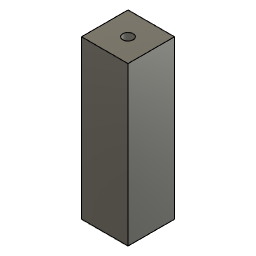
Assembly (Autodesk Fusion 360 archive; units mm, degrees)
design "15*15"
Autodesk Fusion 360 part; units mm, degrees
sketch "Sketch1" plane through (0, 0, 0) normal (0, 1, 0) x (1, 0, 0)
  line L0 (-7.5, 7.5) -> (7.5, 7.5)
  line L1 (-7.5, -7.5) -> (7.5, 7.5) construction
  line L2 (7.5, 7.5) -> (7.5, -7.5)
  circle A0 centre (0, 0) radius 1.7
  line L3 (7.5, -7.5) -> (-7.5, -7.5)
  line L4 (7.5, -7.5) -> (-7.5, 7.5) construction
  line L5 (-7.5, -7.5) -> (-7.5, 7.5)
  dimension "d1" = 15
  dimension "d2" = 15
  dimension "d3" = 3.4
  constraint horizontal L3
  constraint perpendicular L3 L5
  constraint parallel L0 L3
  constraint parallel L2 L5
  constraint coincident A0.centre L4
  constraint coincident A0.centre L1
  constraint coincident A0.centre origin
  measures "d1" distance of L0.start L0.end
  measures "d2" distance of L1.start L0.start
  measures "d3" diameter of A0
extrude "Extrude1" add sketch "Sketch1" along normal blind 5
sketch "Sketch2" plane through (0, 5, 0) normal (0, 1, 0) x (-1, 0, 0)
  circle A0 centre (0, 0) radius 1.7
  line L0 (7.5, 7.5) -> (-7.5, 7.5)
  line L1 (-7.5, 7.5) -> (-7.5, -7.5)
  line L2 (-7.5, -7.5) -> (7.5, -7.5)
  line L3 (7.5, -7.5) -> (7.5, 7.5)
  line L4 (-3.3486, -3.4) -> (-3.3486, 0)
  line L5 (-1.6743, 2.9) -> (-3.3486, 0)
  line L6 (1.6743, 2.9) -> (-1.6743, 2.9)
  circle A1 centre (0, 0) radius 1.7
  line L7 (3.3486, 0) -> (3.3486, -3.1)
  line L8 (3.3486, 0) -> (1.6743, 2.9)
  line L9 (3.3486, -3.1) -> (3.3486, -3.4)
  line L10 (3.3486, -3.4) -> (3.3486, -7.5)
  line L11 (-3.3486, -3.4) -> (-3.3486, -7.5)
  line L12 (3.3486, -7.5) -> (-3.3486, -7.5)
  point P0 (0, 0.15)
  point P1 (0, 0.15)
  dimension "d6" = 2.75
  dimension "d16" = 0.3
  constraint coincident P1 P0
  constraint coincident L2 L10.end
  constraint perpendicular L2 L10
  constraint coincident L2 L11.end
  constraint perpendicular L2 L11
  measures "d6" distance of P1 L6
  measures "d16" distance of L9.end L7.end
extrude "Extrude2" add sketch "Sketch2" along normal blind 4.5 contours L0 L1 L2 L3 L4 L5 L6 L7 L8 L9 L10 L11
sketch "Sketch3" plane through (0, 9.5, 0) normal (0, 1, 0) x (-1, 0, 0)
  line L0 (1.6743, 2.9) -> (3.3486, 0)
  line L1 (3.3486, 0) -> (3.3486, -7.5)
  line L2 (-3.3486, -7.5) -> (-3.3486, 0)
  line L3 (-3.3486, 0) -> (-1.6743, 2.9)
  line L4 (-1.6743, 2.9) -> (1.6743, 2.9)
  line L5 (7.5, -7.5) -> (7.5, 7.5)
  line L6 (7.5, 7.5) -> (-7.5, 7.5)
  line L7 (-7.5, 7.5) -> (-7.5, -7.5)
  line L8 (3.3486, -7.5) -> (7.5, -7.5)
  line L9 (7.5, -7.5) -> (-7.5, -7.5)
  line L10 (-7.5, -7.5) -> (-7.5, 7.5)
  line L11 (-7.5, 7.5) -> (7.5, 7.5)
  line L12 (7.5, 7.5) -> (7.5, -7.5)
  circle A0 centre (0, 0) radius 1.65
  line L13 (-7.5, -7.5) -> (-3.3486, -7.5)
  dimension "d12" = 3.3
  constraint horizontal L9
  constraint vertical L10
  constraint horizontal L11
  constraint vertical L12
  constraint coincident L6.end L7.start
  constraint coincident L5.start L8.end
  constraint coincident A0.centre origin
  measures "d12" diameter of A0
extrude "Extrude3" add sketch "Sketch3" along normal blind 5
sketch "Sketch4" plane through (0, 14.5, 0) normal (0, 1, 0) x (-1, 0, 0)
  circle A0 centre (0, 0) radius 1.65
  line L0 (7.5, 7.5) -> (-7.5, 7.5)
  line L1 (-7.5, 7.5) -> (-7.5, -7.5)
  line L2 (-7.5, -7.5) -> (7.5, -7.5)
  line L3 (7.5, -7.5) -> (7.5, 7.5)
  line L4 (7.5, -7.5) -> (-7.5, -7.5)
  line L5 (-7.5, -7.5) -> (-7.5, 7.5)
  line L6 (-7.5, 7.5) -> (7.5, 7.5)
  line L7 (7.5, 7.5) -> (7.5, -7.5)
  constraint horizontal L4
  constraint vertical L5
  constraint horizontal L6
  constraint vertical L7
  constraint coincident L0.end L1.start
  constraint coincident L2.end L3.start
extrude "Extrude4" add sketch "Sketch4" along normal blind 11 contours A0 | L0 L1 L2 L3 L4 L5 L6 L7
mirror "Mirror1" about plane through (0, 25.5, 0) normal (0, 1, 0) of bodies 1 merged
equation "d6 = ( 5.5 / 2 ) * 1 mm"
equation "d13 = 2.5 mm + 8.5 mm"

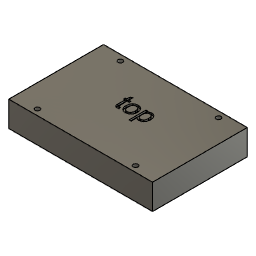
design "RPI"
Autodesk Fusion 360 part; units mm, degrees
sketch "Sketch1" plane through (0, 0, 0) normal (0, 1, 0) x (1, 0, 0)
  line L0 (42.5, -28) -> (-42.5, -28)
  line L1 (-42.5, -28) -> (-42.5, 28)
  line L2 (-42.5, 28) -> (42.5, 28)
  line L3 (42.5, 28) -> (42.5, -28)
  line L4 (42.5, -28) -> (-42.5, 28) construction
  line L5 (-42.5, -28) -> (42.5, 28) construction
  line L6 (0, 28) -> (29, 28)
  line L7 (29, 28) -> (29, -28)
  line L8 (29, 0) -> (29, 24.5)
  line L9 (29, 0) -> (29, -24.5)
  line L10 (29, 24.5) -> (-29, 24.5)
  line L11 (29, -24.5) -> (-29, -24.5)
  circle A0 centre (-29, 24.5) radius 1.4
  circle A1 centre (-29, -24.5) radius 1.4
  circle A2 centre (29, -24.5) radius 1.4
  circle A3 centre (29, 24.5) radius 1.4
  dimension "d1" = 85
  dimension "d2" = 56
  dimension "d3" = 29
  dimension "d4" = 24.5
  dimension "d5" = 24.5
  dimension "d6" = 58
  dimension "d7" = 58
  dimension "d8" = 2.8
  dimension "d9" = 2.8
  dimension "d10" = 2.8
  dimension "d11" = 2.8
  constraint horizontal L0
  constraint perpendicular L0 L1
  constraint parallel L0 L2
  constraint parallel L1 L3
  constraint coincident L4 origin
  constraint coincident L5 origin
  constraint midpoint L2 L6.start
  constraint parallel L2 L6
  constraint coincident L0 L7.end
  constraint perpendicular L0 L7
  constraint midpoint L7 L8.start
  constraint perpendicular L6 L8
  constraint perpendicular L2 L9
  constraint perpendicular L7 L10
  constraint perpendicular L9 L11
  constraint coincident L10.end A0.centre
  constraint coincident L11.end A1.centre
  constraint coincident L9.end L11.start
  constraint coincident L8.end L10.start
  measures "d1" distance of L1.end L2.end
  measures "d2" distance of L0.end L1.end
  measures "d3" distance of L6.start L6.end
  measures "d4" distance of L8.start L8.end
  measures "d5" distance of L8.start L9.end
  measures "d6" distance of L8.end L10.end
  measures "d7" distance of L9.end L11.end
  measures "d8" diameter of A0
  measures "d9" diameter of A1
  measures "d10" diameter of A2
  measures "d11" diameter of A3
extrude "Extrude1" add sketch "Sketch1" along normal blind 15 contours L0 L2 L3 L7 L8 L9 A2 A3 | L0 L1 L2 L6 L7 L8 L9 A2 A3
sketch "Sketch2" plane through (0, 15, 0) normal (0, 1, 0) x (-1, 0, 0)
  circle A0 centre (-29, -24.5) radius 1.4
  circle A1 centre (-29, 24.5) radius 1.4
  circle A2 centre (29, -24.5) radius 1.4
  circle A3 centre (29, 24.5) radius 1.4
  line L0 (-42.5, -28) -> (42.5, -28)
  line L1 (42.5, -28) -> (42.5, 28)
  line L2 (42.5, 28) -> (-42.5, 28)
  line L3 (-42.5, 28) -> (-42.5, -28)
  line L4 (8.6608, -1) -> (-5, -1) construction
  line L5 (-5, -1) -> (-5, -9.5323) construction
  line L6 (-5, -9.5323) -> (8.6608, -9.5323) construction
  line L7 (8.6608, -9.5323) -> (8.6608, -1) construction
  dimension "d14" = 10
  text T0 "top" font "Arial" height 10 align left top in box 13.6608 x 8.5323 at (8.6608, -1) x (-1, 0) y (0, -1) spacing 1 kerned
extrude "Extrude2" cut sketch "Sketch2" against normal blind 1 text T0
equation "d3 = ( 58 / 2 ) * 1 mm"
equation "d4 = ( 49 / 2 ) * 1 mm"
equation "d5 = ( 49 / 2 ) * 1 mm"

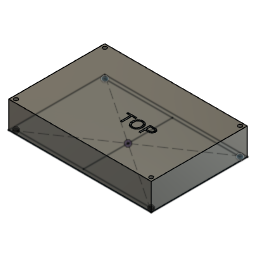
design "AMP"
Autodesk Fusion 360 part; units mm, degrees
sketch "Sketch1" plane through (0, 0, 0) normal (0, 1, 0) x (1, 0, 0)
  line L0 (64.05, -43.15) -> (-64.05, -43.15)
  line L1 (-64.05, -43.15) -> (-64.05, 43.15)
  line L2 (-64.05, 43.15) -> (64.05, 43.15)
  line L3 (64.05, 43.15) -> (64.05, -43.15)
  line L4 (64.05, -43.15) -> (-64.05, 43.15) construction
  line L5 (-64.05, -43.15) -> (64.05, 43.15) construction
  line L6 (-59.3743, 40) -> (-60.75, 40)
  line L7 (59.3743, 40) -> (60.75, 40)
  line L8 (0, 0) -> (0, 39.9)
  line L9 (0, 39.9) -> (60.75, 39.9)
  line L10 (0, 39.9) -> (-60.75, 39.9)
  line L11 (0, 0) -> (0, -39.9)
  line L12 (0, -39.9) -> (-60.75, -39.9)
  line L13 (0, -39.9) -> (60.75, -39.9)
  circle A0 centre (-60.75, -39.9) radius 1.65
  circle A1 centre (60.75, -39.9) radius 1.65
  circle A2 centre (60.75, 40) radius 1.65
  circle A3 centre (-60.75, 40) radius 1.65
  dimension "d1" = 128.1
  dimension "d2" = 86.3
  dimension "d5" = 39.9
  dimension "d6" = 60.75
  dimension "d7" = 60.75
  dimension "d8" = 39.9
  dimension "d9" = 60.75
  dimension "d10" = 60.75
  dimension "d11" = 3.3
  dimension "d12" = 3.3
  dimension "d13" = 3.3
  dimension "d14" = 3.3
  constraint horizontal L0
  constraint perpendicular L0 L1
  constraint parallel L0 L2
  constraint parallel L1 L3
  constraint coincident L4 L8.start
  constraint coincident L5 L8.start
  constraint coincident L8.start L11.start
  constraint parallel L2 L6
  constraint parallel L6 L7
  constraint vertical L8
  constraint perpendicular L8 L9
  constraint perpendicular L8 L10
  constraint coincident L4 L6.start
  constraint coincident L5 L7.start
  constraint vertical L11
  constraint perpendicular L11 L12
  constraint perpendicular L11 L13
  constraint coincident L12.end A0.centre
  constraint coincident L13.end A1.centre
  constraint coincident L7.end A2.centre
  constraint coincident L6.end A3.centre
  measures "d1" distance of L1.end L2.end
  measures "d2" distance of L0.end L1.end
  measures "d5" distance of L8.start L8.end
  measures "d6" distance of L8.end L9.end
  measures "d7" distance of L8.end L10.end
  measures "d8" distance of L8.start L11.end
  measures "d9" distance of L11.end L12.end
  measures "d10" distance of L11.end L13.end
  measures "d11" diameter of A0
  measures "d12" diameter of A1
  measures "d13" diameter of A2
  measures "d14" diameter of A3
extrude "Extrude1" add sketch "Sketch1" along normal blind 24
sketch "Sketch2" plane through (0, 24, 0) normal (0, 1, 0) x (-1, 0, 0)
  circle A0 centre (60.75, 39.9) radius 1.65
  circle A1 centre (-60.75, -40) radius 1.65
  circle A2 centre (-60.75, 39.9) radius 1.65
  circle A3 centre (60.75, -40) radius 1.65
  line L0 (-64.05, -43.15) -> (64.05, -43.15)
  line L1 (64.05, -43.15) -> (64.05, 43.15)
  line L2 (64.05, 43.15) -> (-64.05, 43.15)
  line L3 (-64.05, 43.15) -> (-64.05, -43.15)
  line L4 (0, 15.5213) -> (-15.9408, 15.5213) construction
  line L5 (-15.9408, 15.5213) -> (-15.9408, 0) construction
  line L6 (-15.9408, 0) -> (0, 0) construction
  line L7 (0, 0) -> (0, 15.5213) construction
  dimension "d17" = 10
  text T0 "TOP" font "Arial" height 10 align left top in box 15.9408 x 15.5213 at (0, 15.5213) x (-1, 0) y (0, -1) spacing 1 kerned
  constraint coincident L6.end
extrude "Extrude2" cut sketch "Sketch2" against normal blind 2 text T0
equation "d5 = ( 79.8 / 2 ) * 1 mm"
equation "d8 = ( 79.8 / 2 ) * 1 mm"

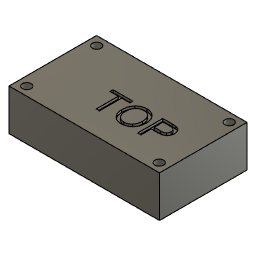
design "Timer relay"
Autodesk Fusion 360 part; units mm, degrees
sketch "Sketch1" plane through (0, 0, 0) normal (0, 1, 0) x (1, 0, 0)
  line L0 (30.1, -17.5) -> (-30.1, -17.5)
  line L1 (-30.1, -17.5) -> (-30.1, 17.5)
  line L2 (-30.1, 17.5) -> (30.1, 17.5)
  line L3 (30.1, 17.5) -> (30.1, -17.5)
  line L4 (30.1, -17.5) -> (-30.1, 17.5) construction
  line L5 (-30.1, -17.5) -> (30.1, 17.5) construction
  line L6 (0, 17.5) -> (-26.5, 17.5)
  line L7 (0, 17.5) -> (26.5, 17.5)
  line L8 (-26.5, 17.5) -> (-26.5, -17.5)
  line L9 (26.5, 17.5) -> (26.5, -17.5)
  line L10 (-26.5, 0) -> (-26.5, 14)
  line L11 (-26.5, 0) -> (-26.5, -14)
  line L12 (26.5, 0) -> (26.5, 14)
  line L13 (26.5, 0) -> (26.5, -14)
  circle A0 centre (-26.5, 14) radius 1.75
  circle A1 centre (26.5, 14) radius 1.75
  circle A2 centre (-26.5, -14) radius 1.75
  circle A3 centre (26.5, -14) radius 1.75
  dimension "d1" = 60.2
  dimension "d2" = 35
  dimension "d3" = 26.5
  dimension "d4" = 26.5
  dimension "d5" = 14
  dimension "d6" = 14
  dimension "d7" = 14
  dimension "d8" = 14
  dimension "d9" = 3.5
  dimension "d10" = 3.5
  dimension "d11" = 3.5
  dimension "d12" = 3.5
  constraint horizontal L0
  constraint perpendicular L0 L1
  constraint parallel L0 L2
  constraint parallel L1 L3
  constraint coincident L4 origin
  constraint coincident L5 origin
  constraint midpoint L2 L6.start
  constraint parallel L2 L6
  constraint parallel L2 L7
  constraint coincident L0 L8.end
  constraint perpendicular L0 L8
  constraint coincident L0 L9.end
  constraint perpendicular L0 L9
  constraint midpoint L8 L10.start
  constraint perpendicular L0 L10
  constraint parallel L8 L11
  constraint midpoint L9 L12.start
  constraint parallel L9 L12
  constraint parallel L9 L13
  constraint coincident L10.end A0.centre
  constraint coincident L12.end A1.centre
  constraint coincident L11.end A2.centre
  constraint coincident L13.end A3.centre
  measures "d1" distance of L1.end L2.end
  measures "d2" distance of L0.end L1.end
  measures "d3" distance of L6.start L6.end
  measures "d4" distance of L6.start L7.end
  measures "d5" distance of L10.start L10.end
  measures "d6" distance of L10.start L11.end
  measures "d7" distance of L12.start L12.end
  measures "d8" distance of L12.start L13.end
  measures "d9" diameter of A0
  measures "d10" diameter of A1
  measures "d11" diameter of A2
  measures "d12" diameter of A3
extrude "Extrude1" add sketch "Sketch1" along normal blind 16.5 contours L0 L2 L3 L9 L12 L13 A1 A3 | L0 L2 L6 L7 L8 L9 L10 L11 L12 L13 A0 A1 A2 A3 | L0 L1 L2 L8 L10 L11 A0 A2
sketch "Sketch2" plane through (0, 16.5, 0) normal (0, 1, 0) x (-1, 0, 0)
  circle A0 centre (26.5, 14) radius 1.75
  circle A1 centre (26.5, -14) radius 1.75
  circle A2 centre (-26.5, 14) radius 1.75
  circle A3 centre (-26.5, -14) radius 1.75
  line L0 (-30.1, -17.5) -> (30.1, -17.5)
  line L1 (30.1, -17.5) -> (30.1, 17.5)
  line L2 (30.1, 17.5) -> (-30.1, 17.5)
  line L3 (-30.1, 17.5) -> (-30.1, -17.5)
  line L4 (8, 8) -> (-13, 8) construction
  line L5 (-13, 8) -> (-13, -2) construction
  line L6 (-13, -2) -> (8, -2) construction
  line L7 (8, -2) -> (8, 8) construction
  dimension "d15" = 10
  text T0 "TOP" font "Arial" height 10 align left top in box 21 x 10 at (8, 8) x (-1, 0) y (0, -1) spacing 1 kerned
extrude "Extrude2" cut sketch "Sketch2" against normal blind 1 text T0
equation "d3 = ( 53 / 2 ) * 1 mm"
equation "d4 = ( 53 / 2 ) * 1 mm"
equation "d5 = ( 28 / 2 ) * 1 mm"
equation "d6 = ( 28 / 2 ) * 1 mm"
equation "d7 = ( 28 / 2 ) * 1 mm"
equation "d8 = ( 28 / 2 ) * 1 mm"

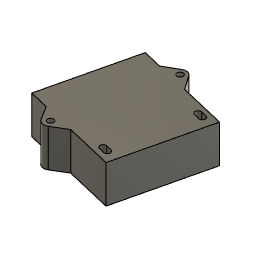
design "buck"
Autodesk Fusion 360 part; units mm, degrees
sketch "Sketch1" plane through (0, 0, 0) normal (0, 1, 0) x (1, 0, 0)
sketch "Sketch2" plane through (0, 0, 0) normal (0, 1, 0) x (1, 0, 0)
  line L0 (-20.092, 27.8314) -> (-31.6, -20.8)
  line L1 (-31.6, -20.8) -> (19.9756, -33.0048)
  line L2 (19.9756, -33.0048) -> (31.4837, 15.6266)
  line L3 (31.4837, 15.6266) -> (-20.092, 27.8314)
  line L4 (24.4539, 11.7249) -> (21.3359, 12.4754)
  line L5 (22.1094, 15.5804) -> (25.144, 14.849)
  arc A0 (22.1094, 15.5804) -> (21.3359, 12.4754) centre (21.7103, 14.031) ccw
  arc A1 (24.3358, 11.7533) -> (25.144, 14.849) centre (24.769, 13.2935) ccw
  arc A2 (14.7267, -28.9815) -> (15.5348, -25.8858) centre (15.1599, -27.4412) ccw
  line L6 (14.8447, -29.0099) -> (11.7267, -28.2593)
  arc A3 (12.5003, -25.1543) -> (11.7267, -28.2593) centre (12.1012, -26.7038) ccw
  line L7 (12.5003, -25.1543) -> (15.5348, -25.8858)
  circle A4 centre (-13.8753, -28.489) radius 1.6
  circle A5 centre (-0.7636, 26.9907) radius 1.6
  line L8 (-10.142, 25.4769) -> (-2.4291, 29.8969)
  line L9 (7.1942, 21.3744) -> (1.9912, 28.8963)
  arc A6 (1.9912, 28.8963) -> (-2.4291, 29.8969) centre (-0.7636, 26.9907) ccw
  line L10 (-21.5261, -23.1839) -> (-17.0355, -30.4438)
  line L11 (-4.4885, -27.2156) -> (-11.9714, -31.6801)
  arc A7 (-17.0355, -30.4438) -> (-11.9714, -31.6801) centre (-13.8753, -28.489) ccw
  dimension "d9" = 53
  dimension "d10" = 3.2
  dimension "d11" = 3.2
  dimension "d12" = 3.2
  dimension "d13" = 3.2
  dimension "d14" = 3.2
  dimension "d15" = 3.2
  constraint perpendicular L0 L1
  constraint parallel L0 L2
  constraint parallel L1 L3
  constraint coincident L4.start A1
  constraint tangent L4 A0
  constraint tangent L5 A1
  constraint coincident L4 A1.start
  constraint coincident L6.start A2
  constraint tangent L6 A3
  constraint tangent A2 L7
  constraint coincident A2.start L6
  constraint coincident L3 L8.start
  constraint coincident L3 L9.start
  constraint concentric A5 A6
  constraint tangent L8 A6
  constraint tangent L9 A6
  constraint coincident L1 L10.start
  constraint coincident L1 L11.start
  constraint concentric A4 A7
  constraint tangent L10 A7
  constraint tangent L11 A7
  measures "d9" distance of L0.start L2.end
  measures "d10" diameter of A0
  measures "d11" diameter of A1
  measures "d12" diameter of A3
  measures "d13" diameter of A2
  measures "d14" diameter of A4
  measures "d15" diameter of A5
extrude "Extrude1" add sketch "Sketch2" along normal blind 20

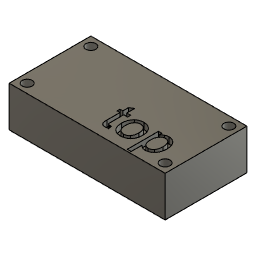
design "Relais"
Autodesk Fusion 360 part; units mm, degrees
sketch "Sketch1" plane through (0, 0, 0) normal (0, 1, 0) x (1, 0, 0)
  line L0 (25.1, -13.15) -> (-25.1, -13.15)
  line L1 (-25.1, -13.15) -> (-25.1, 13.15)
  line L2 (-25.1, 13.15) -> (25.1, 13.15)
  line L3 (25.1, 13.15) -> (25.1, -13.15)
  line L4 (25.1, -13.15) -> (-25.1, 13.15) construction
  line L5 (-25.1, -13.15) -> (25.1, 13.15) construction
  line L6 (0, 0) -> (0, 10.25)
  line L7 (0, 0) -> (0, -10.25)
  line L8 (0, 10.25) -> (-22.2, 10.25)
  line L9 (0, 10.25) -> (22.2, 10.25)
  line L10 (0, -10.25) -> (-22.2, -10.25)
  line L11 (0, -10.25) -> (22.2, -10.25)
  circle A0 centre (-22.2, 10.25) radius 1.6
  circle A1 centre (22.2, 10.25) radius 1.6
  circle A2 centre (-22.2, -10.25) radius 1.6
  circle A3 centre (22.2, -10.25) radius 1.6
  dimension "d1" = 50.2
  dimension "d2" = 26.3
  dimension "d3" = 10.25
  dimension "d4" = 10.25
  dimension "d5" = 22.2
  dimension "d6" = 22.2
  dimension "d7" = 22.2
  dimension "d8" = 22.2
  dimension "d9" = 3.2
  dimension "d10" = 3.2
  dimension "d11" = 3.2
  dimension "d12" = 3.2
  constraint horizontal L0
  constraint perpendicular L0 L1
  constraint parallel L0 L2
  constraint parallel L1 L3
  constraint coincident L4 L6.start
  constraint coincident L5 L6.start
  constraint coincident L6.start L7.start
  constraint perpendicular L2 L6
  constraint parallel L6 L7
  constraint perpendicular L6 L8
  constraint perpendicular L6 L9
  constraint perpendicular L7 L10
  constraint perpendicular L7 L11
  constraint coincident L8.end A0.centre
  constraint coincident L9.end A1.centre
  constraint coincident L10.end A2.centre
  constraint coincident L11.end A3.centre
  measures "d1" distance of L1.end L2.end
  measures "d2" distance of L0.end L1.end
  measures "d3" distance of L6.start L6.end
  measures "d4" distance of L6.start L7.end
  measures "d5" distance of L6.end L8.end
  measures "d6" distance of L6.end L9.end
  measures "d7" distance of L7.end L10.end
  measures "d8" distance of L7.end L11.end
  measures "d9" diameter of A0
  measures "d10" diameter of A1
  measures "d11" diameter of A2
  measures "d12" diameter of A3
extrude "Extrude1" add sketch "Sketch1" along normal blind 13
sketch "Sketch2" plane through (0, 13, 0) normal (0, 1, 0) x (-1, 0, 0)
  circle A0 centre (-22.2, 10.25) radius 1.6
  circle A1 centre (-22.2, -10.25) radius 1.6
  circle A2 centre (22.2, 10.25) radius 1.6
  circle A3 centre (22.2, -10.25) radius 1.6
  line L0 (-25.1, -13.15) -> (25.1, -13.15)
  line L1 (25.1, -13.15) -> (25.1, 13.15)
  line L2 (25.1, 13.15) -> (-25.1, 13.15)
  line L3 (-25.1, 13.15) -> (-25.1, -13.15)
  line L4 (0, 4) -> (-8, 4) construction
  line L5 (-8, 4) -> (-8, 0) construction
  line L6 (-8, 0) -> (0, 0) construction
  line L7 (0, 0) -> (0, 4) construction
  dimension "d15" = 10
  text T0 "top\n" font "Arial" height 10 align left top in box 8 x 4 at (0, 4) x (-1, 0) y (0, -1) spacing 1 kerned
  constraint coincident L6.end
extrude "Extrude2" cut sketch "Sketch2" against normal blind 2 text T0
equation "d3 = ( 20.5 / 2 ) * 1 mm"
equation "d4 = ( 20.5 / 2 ) * 1 mm"
equation "d5 = ( 44.4 / 2 ) * 1 mm"
equation "d6 = ( 44.4 / 2 ) * 1 mm"
equation "d7 = ( 44.4 / 2 ) * 1 mm"
equation "d8 = ( 44.4 / 2 ) * 1 mm"

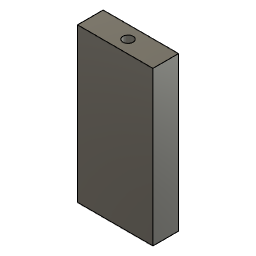
design "20*8.5"
Autodesk Fusion 360 part; units mm, degrees
sketch "Sketch1" plane through (0, 0, 0) normal (0, 1, 0) x (1, 0, 0)
  line L0 (12.5, -4.25) -> (-12.5, -4.25)
  line L1 (-12.5, -4.25) -> (-12.5, 4.25)
  line L2 (-12.5, 4.25) -> (12.5, 4.25)
  line L3 (12.5, 4.25) -> (12.5, -4.25)
  line L4 (12.5, -4.25) -> (-12.5, 4.25) construction
  line L5 (-12.5, -4.25) -> (12.5, 4.25) construction
  circle A0 centre (0, 0) radius 1.7
  dimension "d1" = 25
  dimension "d2" = 8.5
  dimension "d3" = 3.4
  constraint horizontal L0
  constraint perpendicular L0 L1
  constraint parallel L0 L2
  constraint parallel L1 L3
  constraint coincident L4 A0.centre
  constraint coincident L5 A0.centre
  constraint coincident A0.centre origin
  measures "d1" distance of L1.end L2.end
  measures "d2" distance of L0.end L1.end
  measures "d3" diameter of A0
extrude "Extrude1" add sketch "Sketch1" along normal blind 5
sketch "Sketch2" plane through (0, 5, 0) normal (0, 1, 0) x (-1, 0, 0)
  circle A0 centre (0, 0) radius 1.7
  line L0 (-12.5, -4.25) -> (12.5, -4.25)
  line L1 (12.5, -4.25) -> (12.5, 4.25)
  line L2 (12.5, 4.25) -> (-12.5, 4.25)
  line L3 (-12.5, 4.25) -> (-12.5, -4.25)
  line L4 (-1.6743, 2.9) -> (-3.3486, 0)
  line L5 (3.3486, 0) -> (1.6743, 2.9)
  line L6 (1.6743, 2.9) -> (-1.6743, 2.9)
  line L7 (3.3486, 0) -> (3.3486, -2.9)
  line L8 (3.3486, -2.9) -> (3.3486, -3.4)
  line L9 (-3.3486, -3.4) -> (-3.3486, 0)
  line L10 (-3.3486, -3.4) -> (-3.3486, -4.25)
  line L11 (3.3486, -3.4) -> (3.3486, -4.25)
  line L12 (-3.3486, -4.25) -> (3.3486, -4.25)
  dimension "d6" = 2.9
  dimension "d16" = 0.5
  constraint coincident A0.centre origin
  constraint coincident L0 L10.end
  constraint perpendicular L0 L10
  constraint coincident L0 L11.end
  constraint perpendicular L0 L11
  measures "d6" distance of A0.centre L6
  measures "d16" distance of L7.end L8.end
extrude "Extrude2" add sketch "Sketch2" along normal blind 4.5 contours L0 L1 L2 L3 L4 L5 L6 L7 L8 L9 L10 L11
sketch "Sketch3" plane through (0, 9.5, 0) normal (0, 1, 0) x (-1, 0, 0)
  line L0 (-1.6743, 2.9) -> (1.6743, 2.9)
  line L1 (1.6743, 2.9) -> (3.3486, 0)
  line L2 (-3.3486, 0) -> (-1.6743, 2.9)
  line L3 (-12.5, 4.25) -> (-12.5, -4.25)
  line L4 (3.3486, -4.25) -> (12.5, -4.25)
  line L5 (12.5, -4.25) -> (12.5, 4.25)
  line L6 (12.5, 4.25) -> (-12.5, 4.25)
  circle A0 centre (0, 0) radius 1.7
  line L7 (-12.5, 4.25) -> (12.5, 4.25)
  line L8 (12.5, 4.25) -> (12.5, -4.25)
  line L9 (12.5, -4.25) -> (-12.5, -4.25)
  line L10 (-12.5, -4.25) -> (-12.5, 4.25)
  line L11 (-12.5, 4.25) -> (12.5, -4.25) construction
  line L12 (12.5, 4.25) -> (-12.5, -4.25) construction
  line L13 (3.3486, 0) -> (3.3486, -4.25)
  line L14 (-3.3486, -4.25) -> (-3.3486, 0)
  line L15 (-12.5, -4.25) -> (-3.3486, -4.25)
  dimension "d9" = 3.4
  constraint coincident A0.centre origin
  constraint horizontal L7
  constraint perpendicular L7 L8
  constraint parallel L7 L9
  constraint parallel L8 L10
  constraint coincident L11 A0.centre
  constraint coincident L12 A0.centre
  constraint coincident L3.start L6.end
  measures "d9" diameter of A0
extrude "Extrude3" add sketch "Sketch3" along normal blind 5
sketch "Sketch4" plane through (0, 14.5, 0) normal (0, 1, 0) x (-1, 0, 0)
  circle A0 centre (0, 0) radius 1.7
  line L0 (-12.5, -4.25) -> (12.5, -4.25)
  line L1 (12.5, -4.25) -> (12.5, 4.25)
  line L2 (12.5, 4.25) -> (-12.5, 4.25)
  line L3 (-12.5, 4.25) -> (-12.5, -4.25)
  line L4 (-12.5, 4.25) -> (12.5, 4.25)
  line L5 (12.5, 4.25) -> (12.5, -4.25)
  line L6 (12.5, -4.25) -> (-12.5, -4.25)
  line L7 (-12.5, -4.25) -> (-12.5, 4.25)
  line L8 (-12.5, 4.25) -> (12.5, -4.25) construction
  line L9 (12.5, 4.25) -> (-12.5, -4.25) construction
  constraint horizontal L4
  constraint perpendicular L4 L5
  constraint parallel L4 L6
  constraint parallel L5 L7
  constraint coincident L8 A0.centre
  constraint coincident L9 A0.centre
  constraint coincident L2.end L3.start
  constraint coincident A0.centre origin
extrude "Extrude4" add sketch "Sketch4" along normal blind 11 contours A0 | L0 L1 L2 L3 L4 L5 L6 L7
mirror "Mirror1" about plane through (0, 25.5, 0) normal (0, 1, 0) of bodies 1 merged
equation "d6 = ( 5.8 / 2 ) * 1 mm"
equation "d12 = 2.5 mm + 8.5 mm"

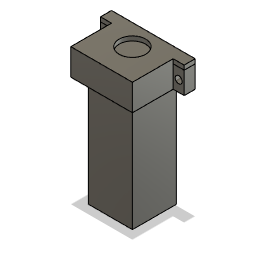
design "holder"
Autodesk Fusion 360 part; units mm, degrees
sketch "Sketch1" plane through (0, 0, 0) normal (0, 1, 0) x (1, 0, 0)
  line L0 (10, -10) -> (-10, -10)
  line L1 (-10, -10) -> (-10, 10)
  line L2 (-10, 10) -> (10, 10)
  line L3 (10, 10) -> (10, -10)
  line L4 (10, -10) -> (-10, 10) construction
  line L5 (-10, -10) -> (10, 10) construction
  dimension "d1" = 20
  dimension "d2" = 20
  constraint horizontal L0
  constraint perpendicular L0 L1
  constraint parallel L0 L2
  constraint parallel L1 L3
  constraint coincident L4 origin
  constraint coincident L5 origin
  measures "d1" distance of L1.end L2.end
  measures "d2" distance of L0.end L1.end
extrude "Extrude1" add sketch "Sketch1" along normal blind 60 makes body 1
sketch "Sketch2" plane through (0, 60, 0) normal (0, 1, 0) x (-1, 0, 0)
  line L0 (-10, -10) -> (10, -10)
  line L1 (10, -10) -> (10, 10)
  line L2 (10, 10) -> (-10, 10)
  line L3 (-10, 10) -> (-10, -10)
  line L4 (14, 14) -> (-14, 14)
  line L5 (-14, 14) -> (-14, -9.5)
  line L6 (14, -9.5) -> (14, 14)
  line L7 (14, -9.5) -> (10, -9.5)
  line L8 (-14, -9.5) -> (-10, -9.5)
  constraint coincident L1 L7.end
  constraint perpendicular L1 L7
  constraint coincident L3 L8.end
  constraint perpendicular L3 L8
extrude "Extrude2" add sketch "Sketch2" against normal blind 10 separate body contours L1 L2 L3 L4 L5 L6 L7 L8 makes body 2
sketch "Sketch3" plane through (-14, 0, 0) normal (-1, 0, 0) x (0, 0, 1)
  line L0 (14, 60) -> (-9.5, 60)
  line L1 (-9.5, 50) -> (14, 50)
  line L2 (14, 50) -> (14, 60)
  line L3 (-9.5, 60) -> (-4.5, 60)
  line L4 (-4.5, 60) -> (-4.5, 50)
  line L5 (-9.5, 60) -> (-9.5, 50)
  dimension "d8" = 5
  constraint coincident L0.end L3.start
  constraint coincident L1 L4.end
  constraint perpendicular L1 L4
  measures "d8" distance of L0.end L3.end
sketch "Sketch4" plane through (14, 0, 0) normal (1, 0, 0) x (0, 0, -1)
  line L0 (9.5, 60) -> (-14, 60)
  line L1 (-14, 60) -> (-14, 50)
  line L2 (-14, 50) -> (9.5, 50)
  line L3 (9.5, 50) -> (9.5, 60)
  line L4 (9.5, 60) -> (4.5, 60)
  line L5 (4.5, 60) -> (4.5, 50)
  dimension "d13" = 5
  constraint coincident L0.start L3.end
  constraint perpendicular L3 L4
  constraint coincident L2 L5.end
  constraint perpendicular L2 L5
  measures "d13" distance of L0.start L4.end
extrude "Extrude3" add sketch "Sketch3" along normal blind 5 contours L0 L1 L3 L4 L5 bodies 1 2
extrude "Extrude4" add sketch "Sketch4" along normal blind 5 contours L0 L2 L3 L4 L5 bodies 2
sketch "Sketch5" plane through (0, 0, -4.5) normal (0, 0, 1) x (1, 0, 0)
  line L0 (14, 60) -> (14, 50)
  line L1 (14, 50) -> (19, 50)
  line L2 (19, 50) -> (19, 60)
  line L3 (19, 60) -> (14, 60)
  line L4 (19, 50) -> (14, 60)
  line L5 (14, 50) -> (19, 60)
  circle A0 centre (16.5, 55) radius 1.6
  dimension "d16" = 3.2
  constraint coincident L1.end L2.start
  constraint coincident L0.start L3.end
  constraint coincident L0.end L1.start
  constraint coincident L2.end L3.start
  constraint midpoint L5 A0.centre
  measures "d16" diameter of A0
sketch "Sketch6" plane through (0, 0, -4.5) normal (0, 0, 1) x (1, 0, 0)
  line L0 (-14, 50) -> (-14, 60)
  line L1 (-14, 60) -> (-19, 60)
  line L2 (-19, 60) -> (-19, 50)
  line L3 (-19, 50) -> (-14, 50)
  line L4 (-14, 50) -> (-19, 60)
  line L5 (-19, 50) -> (-14, 60)
  circle A0 centre (-16.5, 55) radius 1.6
  dimension "d17" = 3.2
  constraint coincident L0.start L3.end
  constraint coincident L1.end L2.start
  constraint coincident L2.end L3.start
  constraint coincident L0.end L1.start
  constraint midpoint L4 A0.centre
  measures "d17" diameter of A0
extrude "Extrude5" cut sketch "Sketch5" against normal blind 8 contours L4 L5 A0 | L4 L5 A0 | L4 L5 A0 | L4 L5 A0 bodies 2
extrude "Extrude6" cut sketch "Sketch6" against normal blind 11 contours L4 L5 A0 | L4 L5 A0 | L4 L5 A0 | L4 L5 A0 bodies 2
copy_body "CopyPasteBodies1" bodies 2 makes body 3
move_body "Move1" bodies 3 to x (1, 0, 0) y (0, 1, 0) z (0, 0, 1) at (0, -50, 0)
sketch "Sketch7" plane through (0, 60, 0) normal (0, 1, 0) x (-1, 0, 0)
  line L0 (14, -4.5) -> (14, 14)
  line L1 (14, 14) -> (-14, 14)
  line L2 (-14, 14) -> (-14, -4.5)
  line L3 (-14, -4.5) -> (-19, -4.5)
  line L4 (-19, -4.5) -> (-19, -9.5)
  line L5 (-19, -9.5) -> (-14, -9.5)
  line L6 (-14, -9.5) -> (-10, -9.5)
  line L7 (-10, -9.5) -> (-10, 10)
  line L8 (-10, 10) -> (10, 10)
  line L9 (10, 10) -> (10, -9.5)
  line L10 (10, -9.5) -> (14, -9.5)
  line L11 (14, -9.5) -> (19, -9.5)
  line L12 (19, -9.5) -> (19, -4.5)
  line L13 (19, -4.5) -> (14, -4.5)
  circle A0 centre (0, 0) radius 6
  line L14 (14, -9.5) -> (-14, -9.5)
  line L15 (-14, -4.5) -> (-14, 14)
  line L16 (-14, 14) -> (14, 14)
  line L17 (14, 14) -> (14, -4.5)
  line L18 (19, -9.5) -> (14, -9.5)
  line L19 (14, -4.5) -> (19, -4.5)
  line L20 (19, -4.5) -> (19, -9.5)
  line L21 (-14, -9.5) -> (-19, -9.5)
  line L22 (-19, -9.5) -> (-19, -4.5)
  line L23 (-19, -4.5) -> (-14, -4.5)
  line L24 (-14, -4.5) -> (-14, -9.5)
  dimension "d22" = 12
  constraint coincident A0.centre origin
  constraint horizontal L14
  constraint vertical L15
  constraint horizontal L16
  constraint vertical L17
  constraint coincident L1.end L2.start
  constraint coincident L10.end L11.start
  constraint horizontal L18
  constraint horizontal L19
  constraint vertical L20
  constraint coincident L0.start L13.end
  constraint coincident L11.end L12.start
  constraint horizontal L21
  constraint vertical L22
  constraint horizontal L23
  constraint vertical L24
  constraint coincident L3.end L4.start
  measures "d22" diameter of A0
extrude "Extrude7" add sketch "Sketch7" along normal blind 2 bodies 2
hidden bodies 3

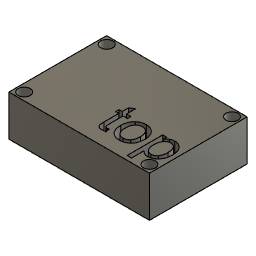
design "CANSHIELD"
Autodesk Fusion 360 part; units mm, degrees
sketch "Sketch1" plane through (0, 0, 0) normal (0, 1, 0) x (1, 0, 0)
  line L0 (19.8, -13.75) -> (-19.8, -13.75)
  line L1 (-19.8, -13.75) -> (-19.8, 13.75)
  line L2 (-19.8, 13.75) -> (19.8, 13.75)
  line L3 (19.8, 13.75) -> (19.8, -13.75)
  line L4 (19.8, -13.75) -> (-19.8, 13.75) construction
  line L5 (-19.8, -13.75) -> (19.8, 13.75) construction
  line L6 (0, 0) -> (0, 11.65)
  line L7 (0, 0) -> (0, -11.6)
  line L8 (0, -11.6) -> (-17.65, -11.6)
  line L9 (0, -11.6) -> (17.65, -11.6)
  line L10 (0, 11.65) -> (-17.65, 11.65)
  line L11 (0, 11.65) -> (17.65, 11.65)
  circle A0 centre (-17.65, 11.65) radius 1.7
  circle A1 centre (17.65, 11.65) radius 1.7
  circle A2 centre (-17.65, -11.6) radius 1.7
  circle A3 centre (17.65, -11.6) radius 1.7
  dimension "d1" = 39.6
  dimension "d2" = 27.5
  dimension "d3" = 11.65
  dimension "d4" = 11.6
  dimension "d5" = 17.65
  dimension "d6" = 17.65
  dimension "d7" = 17.65
  dimension "d8" = 17.65
  dimension "d9" = 3.4
  dimension "d10" = 3.4
  dimension "d11" = 3.4
  dimension "d12" = 3.4
  constraint horizontal L0
  constraint perpendicular L0 L1
  constraint parallel L0 L2
  constraint parallel L1 L3
  constraint coincident L4 L6.start
  constraint coincident L5 L6.start
  constraint coincident L6.start L7.start
  constraint vertical L6
  constraint parallel L6 L7
  constraint perpendicular L7 L8
  constraint perpendicular L7 L9
  constraint perpendicular L6 L10
  constraint perpendicular L6 L11
  constraint coincident L10.end A0.centre
  constraint coincident L11.end A1.centre
  constraint coincident L8.end A2.centre
  constraint coincident L9.end A3.centre
  measures "d1" distance of L1.end L2.end
  measures "d2" distance of L0.end L1.end
  measures "d3" distance of L6.start L6.end
  measures "d4" distance of L6.start L7.end
  measures "d5" distance of L7.end L8.end
  measures "d6" distance of L7.end L9.end
  measures "d7" distance of L6.end L10.end
  measures "d8" distance of L6.end L11.end
  measures "d9" diameter of A0
  measures "d10" diameter of A1
  measures "d11" diameter of A2
  measures "d12" diameter of A3
extrude "Extrude1" add sketch "Sketch1" along normal blind 11.5
sketch "Sketch2" plane through (0, 11.5, 0) normal (0, 1, 0) x (-1, 0, 0)
  circle A0 centre (-17.65, 11.6) radius 1.7
  circle A1 centre (17.65, -11.65) radius 1.7
  circle A2 centre (-17.65, -11.65) radius 1.7
  circle A3 centre (17.65, 11.6) radius 1.7
  line L0 (-19.8, -13.75) -> (19.8, -13.75)
  line L1 (19.8, -13.75) -> (19.8, 13.75)
  line L2 (19.8, 13.75) -> (-19.8, 13.75)
  line L3 (-19.8, 13.75) -> (-19.8, -13.75)
  line L4 (0, 5) -> (-13, 5) construction
  line L5 (-13, 5) -> (-13, 0) construction
  line L6 (-13, 0) -> (0, 0) construction
  line L7 (0, 0) -> (0, 5) construction
  dimension "d15" = 10
  text T0 "top\n" font "Arial" height 10 align left top in box 13 x 5 at (0, 5) x (-1, 0) y (0, -1) spacing 1 kerned
  constraint coincident L6.end
extrude "Extrude2" cut sketch "Sketch2" against normal blind 5 text T0
equation "d3 = ( 23.3 / 2 ) * 1 mm"
equation "d4 = ( 23.2 / 2 ) * 1 mm"
equation "d5 = ( 35.3 / 2 ) * 1 mm"
equation "d6 = ( 35.3 / 2 ) * 1 mm"
equation "d7 = ( 35.3 / 2 ) * 1 mm"
equation "d8 = ( 35.3 / 2 ) * 1 mm"

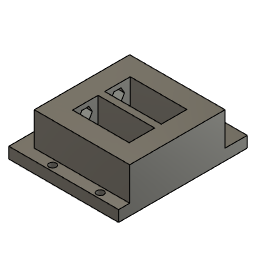
design "ISO connector"
Autodesk Fusion 360 part; units mm, degrees
sketch "Sketch2" plane through (0, 0, 0) normal (0, 1, 0) x (1, 0, 0)
  line L0 (12.75, 13) -> (-12.75, 13)
  line L1 (-12.75, 13) -> (-12.75, -13)
  line L2 (-12.75, -13) -> (12.75, -13)
  line L3 (12.75, -13) -> (12.75, 13)
  line L4 (12.75, 13) -> (-12.75, -13) construction
  line L5 (-12.75, 13) -> (12.75, -13) construction
  line L6 (-12.75, -13) -> (-12.75, -1.5)
  line L7 (-12.75, 13) -> (-12.75, 1.5)
  line L8 (-12.75, 1.5) -> (12.75, 1.5)
  line L9 (-12.75, -1.5) -> (12.75, -1.5)
  line L10 (21.5, -21.5) -> (-21.5, -21.5)
  line L11 (-21.5, -21.5) -> (-21.5, 21.5)
  line L12 (-21.5, 21.5) -> (21.5, 21.5)
  line L13 (21.5, 21.5) -> (21.5, -21.5)
  line L14 (21.5, -21.5) -> (-21.5, 21.5) construction
  line L15 (-21.5, -21.5) -> (21.5, 21.5) construction
  line L16 (-21.5, -21.5) -> (-21.5, -26.5)
  line L17 (21.5, -21.5) -> (21.5, -26.5)
  line L18 (21.5, -26.5) -> (-21.5, -26.5)
  line L19 (-21.5, -26.5) -> (-28, -26.5)
  line L20 (-28, -26.5) -> (-28, 21.5)
  line L21 (-28, 21.5) -> (-21.5, 21.5)
  line L22 (-28, 21.5) -> (-28, 31.5)
  line L23 (-28, 31.5) -> (21.5, 31.5)
  line L24 (21.5, 31.5) -> (21.5, 21.5)
  line L25 (-21.5, -24) -> (21.5, -24)
  line L26 (-21.5, -24) -> (0, -24)
  line L27 (0, -24) -> (21.5, -24)
  circle A0 centre (-10.75, -24) radius 1.6
  circle A1 centre (10.75, -24) radius 1.6
  line L28 (-24.75, -26.5) -> (-24.75, 21.5)
  line L29 (-24.75, -2.5) -> (-28, -2.5)
  line L30 (-24.75, -2.5) -> (-24.75, 21.5)
  line L31 (-24.75, -2.5) -> (-24.75, -26.5)
  circle A2 centre (-24.75, 9.5) radius 1.6
  circle A3 centre (-24.75, -14.5) radius 1.6
  line L32 (-28, 26.5) -> (21.5, 26.5)
  line L33 (-3.25, 31.5) -> (-3.25, 26.5)
  line L34 (-28, 26.5) -> (-3.25, 26.5)
  line L35 (-3.25, 26.5) -> (21.5, 26.5)
  circle A4 centre (-15.625, 26.5) radius 1.6
  circle A5 centre (9.125, 26.5) radius 1.6
  dimension "d10" = 25.5
  dimension "d11" = 26
  dimension "d12" = 11.5
  dimension "d13" = 11.5
  dimension "d14" = 43
  dimension "d15" = 43
  dimension "d16" = 5
  dimension "d17" = 5
  dimension "d18" = 6.5
  dimension "d19" = 10
  dimension "d20" = 3.2
  dimension "d21" = 3.2
  dimension "d23" = 3.2
  dimension "d24" = 3.2
  dimension "d25" = 3.2
  dimension "d26" = 3.2
  constraint horizontal L0
  constraint perpendicular L0 L1
  constraint parallel L0 L2
  constraint parallel L1 L3
  constraint coincident L4 origin
  constraint coincident L5 origin
  constraint perpendicular L2 L6
  constraint perpendicular L0 L7
  constraint coincident L3 L8.end
  constraint perpendicular L3 L8
  constraint coincident L3 L9.end
  constraint perpendicular L3 L9
  constraint horizontal L10
  constraint perpendicular L10 L11
  constraint parallel L10 L12
  constraint parallel L11 L13
  constraint coincident L14 origin
  constraint coincident L15 origin
  constraint perpendicular L10 L16
  constraint perpendicular L10 L17
  constraint perpendicular L16 L19
  constraint perpendicular L12 L20
  constraint perpendicular L11 L21
  constraint perpendicular L21 L22
  constraint perpendicular L13 L23
  constraint perpendicular L12 L24
  constraint midpoint L16 L25.start
  constraint midpoint L17 L25.end
  constraint midpoint L25 L26.end
  constraint midpoint L26 A0.centre
  constraint midpoint L27 A1.centre
  constraint midpoint L19 L28.start
  constraint midpoint L21 L28.end
  constraint midpoint L28 L29.start
  constraint midpoint L20 L29.end
  constraint midpoint L30 A2.centre
  constraint midpoint L31 A3.centre
  constraint midpoint L22 L32.start
  constraint midpoint L24 L32.end
  constraint midpoint L23 L33.start
  constraint midpoint L32 L33.end
  constraint midpoint L34 A4.centre
  constraint midpoint L35 A5.centre
  measures "d10" distance of L1.end L2.end
  measures "d11" distance of L0.end L1.end
  measures "d12" distance of L1.end L6.end
  measures "d13" distance of L0.end L7.end
  measures "d14" distance of L11.end L12.end
  measures "d15" distance of L10.end L11.end
  measures "d16" distance of L10.end L16.end
  measures "d17" distance of L10.start L17.end
  measures "d18" distance of L16.end L19.end
  measures "d19" distance of L20.end L22.end
  measures "d20" diameter of A0
  measures "d21" diameter of A1
  measures "d23" diameter of A2
  measures "d24" diameter of A3
  measures "d25" diameter of A4
  measures "d26" diameter of A5
extrude "Extrude2" add sketch "Sketch2" along normal blind 5 contours L10 L16 L17 L25 L26 L27 A0 A1 | L11 L16 L19 L21 L28 L30 L31 A2 A3 | L12 L21 L22 L24 L32 L34 L35 A4 A5 | L16 L17 L18 L25 L26 L27 A0 A1 | L23 L24 L32 L33 L35 A5 | L20 L21 L28 L29 L30 A2 | L19 L20 L28 L29 L31 A3 | L22 L23 L32 L33 L34 A4
extrude "Extrude3" add sketch "Sketch2" along normal blind 20 contours L1 L3 L8 L9 | L10 L11 L12 L13
sketch "Sketch3" plane through (0, 0, 0) normal (0, 0, 1) x (1, 0, 0)
sketch "Sketch4" plane through (-12.75, 0, 0) normal (1, 0, 0) x (0, 0, -1)
  line L0 (-13, 0) -> (-1.5, 0)
  line L1 (-1.5, 0) -> (-1.5, 20)
  line L2 (-1.5, 20) -> (-13, 20)
  line L3 (-13, 20) -> (-13, 0)
  line L4 (-7.25, 20) -> (-7.25, 15)
  line L5 (-5.6623, 12.25) -> (-4.0746, 15)
  line L6 (-4.0746, 15) -> (-5.6623, 17.75)
  line L7 (-5.6623, 17.75) -> (-8.8377, 17.75)
  line L8 (-8.8377, 17.75) -> (-10.4254, 15)
  line L9 (-10.4254, 15) -> (-8.8377, 12.25)
  line L10 (-8.8377, 12.25) -> (-5.6623, 12.25)
  circle A0 centre (-7.25, 15) radius 1.6
  point P0 (-7.25, 15)
  dimension "d31" = 5
  dimension "d32" = 2.75
  dimension "d33" = 3.2
  constraint midpoint L2 L4.start
  constraint perpendicular L2 L4
  constraint coincident P0 L4.end
  measures "d31" distance of L4.start P0
  measures "d32" distance of P0 L10
  measures "d33" diameter of A0
sketch "Sketch5" plane through (-12.75, 0, 0) normal (1, 0, 0) x (0, 0, -1)
  line L0 (1.5, 0) -> (13, 0)
  line L1 (13, 0) -> (13, 20)
  line L2 (13, 20) -> (1.5, 20)
  line L3 (1.5, 20) -> (1.5, 0)
  line L4 (5.6623, 12.25) -> (8.8377, 12.25)
  line L5 (7.25, 20) -> (7.25, 15)
  line L6 (4.0746, 15) -> (5.6623, 12.25)
  circle A0 centre (7.25, 15) radius 1.6
  line L7 (10.4254, 15) -> (8.8377, 17.75)
  line L8 (8.8377, 12.25) -> (10.4254, 15)
  line L9 (5.6623, 17.75) -> (4.0746, 15)
  line L10 (8.8377, 17.75) -> (5.6623, 17.75)
  point P0 (7.25, 15)
  dimension "d38" = 5
  dimension "d39" = 2.75
  dimension "d40" = 3.2
  constraint coincident P0 L5.end
  measures "d38" distance of L5.start P0
  measures "d39" distance of P0 L4
  measures "d40" diameter of A0
extrude "Extrude4" cut sketch "Sketch5" sketch "Sketch4" against normal blind 4.3 contours L4 L6 L7 L8 L9 L10 | A0 of sketch 2 contours L5 L6 L7 L8 L9 L10 | A0
extrude "Extrude5" cut sketch "Sketch5" sketch "Sketch4" against normal blind 17 contours A0 of sketch 2 contours A0
equation "d32 = ( 5.5 / 2 ) * 1 mm"
equation "d39 = ( 5.5 / 2 ) * 1 mm"
